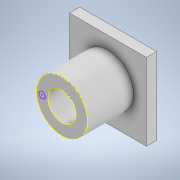
# Autodesk Inventor part: MotorDemoV1
Saved by Autodesk Inventor 2020 (Build 240168000, 168)
## iProperties
Created: 2023-01-12
Part Number: MotorDemoV1
Material: Generic
Document SubType Name: Modeling
Designer: agraa4529
Density: 1 g/cm^3
Appearance: Default
Author: agraa4529
Autodesk Inventor part; units mm, degrees
ref_plane "YZ Plane" through (0, 0, 0) normal (1, 0, 0) x (0, 1, 0)
ref_plane "XZ Plane" through (0, 0, 0) normal (0, 1, 0) x (-1, 0, 0)
ref_plane "XY Plane" through (0, 0, 0) normal (0, 0, 1) x (1, 0, 0)
sketch "Sketch1" plane through (0, 0, 0) normal (0, 0, 1) x (1, 0, 0)
  circle A0 centre (0, 0) radius 5.5
  circle A1 centre (0, 0) radius 10
  dimension "d0" = 11
  dimension "d1" = 20
  constraints: 2 centre point, 2 coincident
  measures "d0" diameter of A0
  measures "d1" diameter of A1
extrude "Extrusion1" add sketch "Sketch1" along normal blind 18
sketch "Sketch3" plane through (0, 0, 0) normal (0, 0, -1) x (-1, 0, 0)
  line L0 (15, -15) -> (-15, -15)
  line L1 (-15, -15) -> (-15, 15)
  line L2 (-15, 15) -> (15, 15)
  line L3 (15, 15) -> (15, -15)
  line L4 (15, -15) -> (-15, 15) construction
  line L5 (-15, -15) -> (15, 15) construction
  point P0 (0, 0)
  dimension "d4" = 30
  dimension "d5" = 30
  constraints: 12 end point, 2 midpoint, 2 parallel, 1 horizontal, 1 perpendicular
  measures "d4" distance of L0.end L1.end
  measures "d5" distance of L0.start L0.end
extrude "Extrusion2" add sketch "Sketch3" along normal blind 4
sketch "Sketch5" plane through (0, 0, 0) normal (0, 0, 1) x (1, 0, 0)
  line L0 (-3, 3) -> (3, 3)
  line L1 (3, 3) -> (3, -3)
  line L2 (3, -3) -> (-3, -3)
  line L3 (-3, -3) -> (-3, 3)
  line L4 (-3, 3) -> (3, -3) construction
  line L5 (3, 3) -> (-3, -3) construction
  point P0 (0, 0)
  dimension "d8" = 6
  dimension "d9" = 6
  constraints: 12 end point, 2 midpoint, 2 parallel, 1 horizontal, 1 perpendicular
  measures "d8" distance of L1.end L2.end
  measures "d9" distance of L0.end L1.end
extrude "Extrusion3" cut sketch "Sketch5" against normal blind 10
sketch "Sketch6" plane through (0, 0, 18) normal (0, 0, 1) x (1, 0, 0)
  circle A0 centre (0, 0) radius 10 projected
  line L0 (-10, 0) -> (-5.5, 0) construction
  circle A1 centre (0, 0) radius 5.5 projected
  circle A2 centre (-7.75, 0) radius 1.244
  constraints: 2 end point, 2 horizontal alignment, 1 centre point, 1 horizontal, 1 midpoint, 2 other
body "Solid1"
